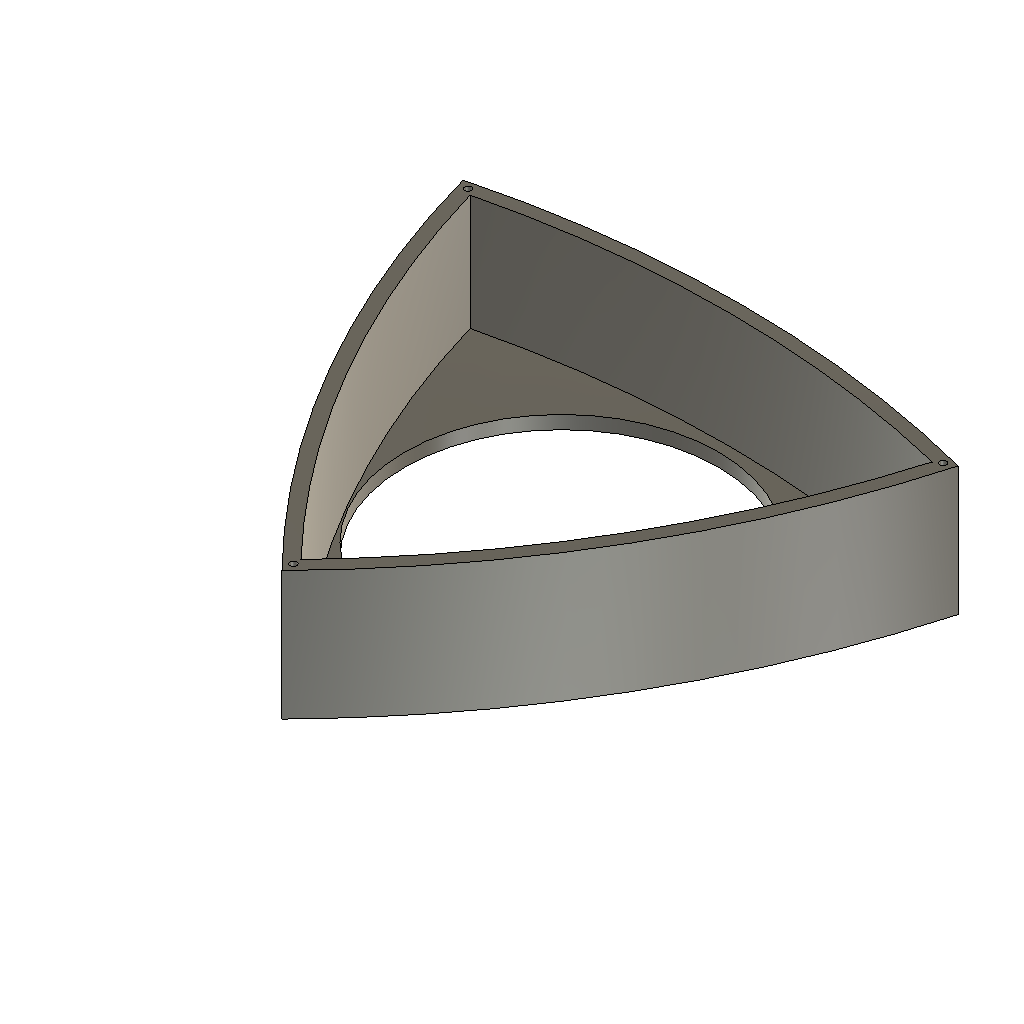
Case (Autodesk Fusion 360 design; units mm, degrees)
Autodesk Fusion 360 part; units mm, degrees
sketch "Base" plane through (0, 0, 0) normal (0, 0, 1) x (1, 0, 0)
  line L0 (0, 0) -> (150, 0)
  line L1 (0, 0) -> (75, -129.9038)
  line L2 (0, 0) -> (150, 0) construction
  line L3 (75, -129.9038) -> (150, 0)
  arc A0 (150, 0) -> (0, 0) centre (75, -290.4738) ccw
  arc A1 (75, -129.9038) -> (150, 0) centre (-139.0576, 80.285) ccw
  arc A2 (0, 0) -> (75, -129.9038) centre (289.0576, 80.285) ccw
  dimension "d1" = 150
  dimension "d3" = 60
  dimension "d4" = 150
  dimension "d5" = 300
  dimension "d7" = 300
  dimension "d8" = 300
  constraint coincident L0.start L1.start
  constraint horizontal L0
  constraint horizontal L2
  measures "d1" distance of L0.start L0.end
  measures "d3" angle of L1 L2
  measures "d4" distance of L0.start L1.end
  measures "d5" radius of A0
  measures "d7" radius of A1
  measures "d8" radius of A2
extrude "Extrude1" add sketch "Base" along normal blind 4
sketch "Walls" plane through (0, 0, 4) normal (0, 0, 1) x (-1, 0, 0)
  arc A0 (0, 0) -> (-75, 129.9038) centre (-289.0576, -80.285) ccw
  arc A1 (-75, 129.9038) -> (-150, 0) centre (139.0576, -80.285) ccw
  arc A2 (-150, 0) -> (0, 0) centre (-75, 290.4738) ccw
  arc A3 (-75, 124.1541) -> (-145.0206, 2.8749) centre (139.0576, -80.285) ccw
  arc A4 (-145.0206, 2.8749) -> (-4.9794, 2.8749) centre (-75, 290.4738) ccw
  arc A5 (-4.9794, 2.8749) -> (-75, 124.1541) centre (-289.0576, -80.285) ccw
  dimension "d11" = -4
extrude "Extrude2" add sketch "Walls" along normal blind 35
sketch "Cutout" plane through (0, 0, 4) normal (0, 0, 1) x (-1, 0, 0)
  arc A0 (-75, 124.1541) -> (-145.0206, 2.8749) centre (139.0576, -80.285) ccw
  arc A1 (-145.0206, 2.8749) -> (-4.9794, 2.8749) centre (-75, 290.4738) ccw
  arc A2 (-4.9794, 2.8749) -> (-75, 124.1541) centre (-289.0576, -80.285) ccw
  circle A3 centre (-75, 45.1538) radius 47.5
  point P0 (-75, 129.9038)
  dimension "d14" = 95
  dimension "d16" = 84.75
  dimension "d17" = 75
  measures "d14" diameter of A3
  measures "d16" vertical distance of A3.centre P0
  measures "d17" horizontal distance of origin A3.centre
extrude "Extrude3" cut sketch "Cutout" against normal blind 4 contours A3
sketch "Screw holes" plane through (0, 0, 39) normal (0, 0, 1) x (-1, 0, 0)
  arc A0 (-4.9794, 2.8749) -> (-75, 124.1541) centre (-289.0576, -80.285) ccw
  arc A1 (-145.0206, 2.8749) -> (-4.9794, 2.8749) centre (-75, 290.4738) ccw
  arc A2 (-75, 124.1541) -> (-145.0206, 2.8749) centre (139.0576, -80.285) ccw
  arc A3 (-150, 0) -> (0, 0) centre (-75, 290.4738) ccw
  arc A4 (0, 0) -> (-75, 129.9038) centre (-289.0576, -80.285) ccw
  arc A5 (-75, 129.9038) -> (-150, 0) centre (139.0576, -80.285) ccw
  circle A6 centre (-3, 1.5) radius 1
  circle A7 centre (-147, 1.5) radius 1
  circle A8 centre (-75, 126.4038) radius 1
  dimension "d20" = 2
  dimension "d22" = 1.5
  dimension "d23" = 3
  dimension "d24" = 2
  dimension "d25" = 1.5
  dimension "d26" = 3
  dimension "d27" = 2
  dimension "d28" = 3.5
  measures "d20" diameter of A6
  measures "d22" vertical distance of A3.end A6.centre
  measures "d23" horizontal distance of A3.end A6.centre
  measures "d24" diameter of A7
  measures "d25" vertical distance of A3.start A7.centre
  measures "d26" horizontal distance of A3.start A7.centre
  measures "d27" diameter of A8
  measures "d28" distance of A4.end A8.centre
extrude "Extrude4" cut sketch "Screw holes" against normal blind 5 contours A6 | A7 | A8
